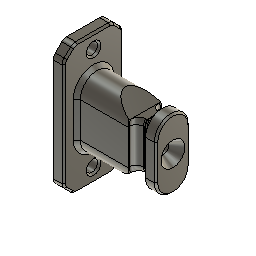
SKADIS_BackSupports (Autodesk Fusion 360 design; units mm, degrees)
Autodesk Fusion 360 part; units mm, degrees
sketch "SlotLayout" plane through (0, 0, 0) normal (1, 0, 0) x (0, 1, 0)
  line L0 (-22.4, 25) -> (-22.4, 15)
  line L1 (82.4, 5) -> (82.4, -5)
  line L2 (-37.6, -5) -> (-37.6, 5)
  line L3 (-80, 5) -> (-80, -5) construction
  line L4 (-97.6, 15) -> (-97.6, 25)
  line L5 (2.4, -5) -> (2.4, 5)
  arc A0 (-77.6, 5) -> (-82.4, 5) centre (-80, 5) ccw
  arc A1 (22.4, 25) -> (17.6, 25) centre (20, 25) ccw
  arc A2 (-97.6, 25) -> (-102.4, 25) centre (-100, 25) ccw
  arc A3 (97.6, 15) -> (102.4, 15) centre (100, 15) ccw
  line L6 (-60, 25) -> (-60, 15) construction
  line L7 (-77.6, -5) -> (-77.6, 5)
  arc A4 (77.6, -5) -> (82.4, -5) centre (80, -5) ccw
  line L8 (-40, 5) -> (-40, -5) construction
  line L9 (-57.6, 15) -> (-57.6, 25)
  line L10 (-62.4, 25) -> (-62.4, 15)
  line L11 (-102.4, 25) -> (-102.4, 15)
  line L12 (97.6, 15) -> (97.6, 25)
  arc A5 (-102.4, 15) -> (-97.6, 15) centre (-100, 15) ccw
  line L13 (20, 25) -> (20, 15) construction
  line L14 (22.4, 25) -> (22.4, 15)
  line L15 (-80, 0) -> (0, 0) construction
  line L16 (62.4, 25) -> (62.4, 15)
  line L17 (42.4, 5) -> (42.4, -5)
  arc A6 (2.5, 5) -> (-2.5, 5) centre (0, 5) ccw
  arc A7 (2.4, 5) -> (-2.4, 5) centre (0, 5) ccw
  line L18 (80, 5) -> (80, -5) construction
  arc A8 (82.4, 5) -> (77.6, 5) centre (80, 5) ccw
  arc A9 (-2.5, -5) -> (2.5, -5) centre (0, -5) ccw
  arc A10 (57.6, 15) -> (62.4, 15) centre (60, 15) ccw
  arc A11 (62.4, 25) -> (57.6, 25) centre (60, 25) ccw
  line L19 (17.6, 15) -> (17.6, 25)
  line L20 (-20, 25) -> (-20, 15) construction
  line L21 (-42.4, 5) -> (-42.4, -5)
  line L22 (60, 25) -> (60, 15) construction
  arc A12 (42.4, 5) -> (37.6, 5) centre (40, 5) ccw
  line L23 (-100, 25) -> (-100, 15) construction
  line L24 (100, 25) -> (100, 15) construction
  arc A13 (-57.6, 25) -> (-62.4, 25) centre (-60, 25) ccw
  arc A14 (37.6, -5) -> (42.4, -5) centre (40, -5) ccw
  line L25 (40, 5) -> (40, -5) construction
  line L26 (-17.6, 15) -> (-17.6, 25)
  arc A15 (-17.6, 25) -> (-22.4, 25) centre (-20, 25) ccw
  line L27 (-82.4, 5) -> (-82.4, -5)
  line L28 (-2.5, 5) -> (-2.5, -5)
  line L29 (-2.4, 5) -> (-2.4, -5)
  line L30 (102.4, 25) -> (102.4, 15)
  arc A16 (17.6, 15) -> (22.4, 15) centre (20, 15) ccw
  arc A17 (-22.4, 15) -> (-17.6, 15) centre (-20, 15) ccw
  line L31 (37.6, -5) -> (37.6, 5)
  line L32 (0, 5) -> (0, -5) construction
  arc A18 (-62.4, 15) -> (-57.6, 15) centre (-60, 15) ccw
  arc A19 (-42.4, -5) -> (-37.6, -5) centre (-40, -5) ccw
  arc A20 (-2.4, -5) -> (2.4, -5) centre (0, -5) ccw
  arc A21 (102.4, 25) -> (97.6, 25) centre (100, 25) ccw
  arc A22 (-82.4, -5) -> (-77.6, -5) centre (-80, -5) ccw
  arc A23 (-37.6, 5) -> (-42.4, 5) centre (-40, 5) ccw
  line L33 (77.6, -5) -> (77.6, 5)
  line L34 (57.6, 15) -> (57.6, 25)
  line L35 (2.5, -5) -> (2.5, 5)
  point P0 (-20, 20)
  point P1 (-40, 0)
  dimension "d9" = -40
  dimension "d10" = 0
  dimension "d255" = 0.1
  dimension "d22" = 10
  dimension "d23" = 2.4
  dimension "d4" = 40
  dimension "d25" = 40
  dimension "d26" = 20
  dimension "d27" = 20
  constraint tangent L27 A22
  constraint tangent L7 A22
  constraint parallel L7 L27
  constraint tangent A0 L7
  constraint tangent A0 L27
  constraint vertical L3
  constraint tangent L21 A19
  constraint tangent L2 A19
  constraint parallel L2 L21
  constraint tangent L2 A23
  constraint tangent L21 A23
  constraint vertical L8
  constraint tangent L29 A20
  constraint tangent L5 A20
  constraint parallel L5 L29
  constraint tangent L5 A7
  constraint tangent A7 L29
  constraint parallel L2 L32
  constraint midpoint L15.start L3
  constraint midpoint L15.end L32
  constraint horizontal L15
  constraint equal L8 L32
  constraint equal L3 L8
  constraint midpoint P1 L8
  constraint coincident P1 L15
  constraint equal A7 A23
  constraint equal A0 A23
  constraint coincident L15.end origin
  constraint symmetric A0.end L1.start L32
  constraint symmetric L1.end L27.end L32
  constraint symmetric L7.start A4.start L32
  constraint symmetric A8.end A0.start L32
  constraint symmetric A4 L32 A22
  constraint symmetric A0 A8 L32
  constraint symmetric L17.start L21.start L32
  constraint symmetric L17.end L21.end L32
  constraint symmetric A14.start L2.start L32
  constraint symmetric A12.end L2.end L32
  constraint symmetric A14 L32 A19
  constraint symmetric A12 L32 A23
  constraint tangent L0 A17
  constraint tangent L26 A17
  constraint parallel L0 L26
  constraint tangent L26 A15
  constraint tangent L0 A15
  constraint vertical L20
  constraint equal L20 L32
  constraint equal A7 A15
  constraint midpoint P0 L20
  constraint symmetric L0.end L14.end L32
  constraint symmetric L26.end A1.end L32
  constraint symmetric L0.start A1.start L32
  constraint symmetric L26.start L19.start L32
  constraint symmetric A1 A15 L32
  constraint symmetric A16 A17 L32
  constraint symmetric A11.end L9.end L32
  constraint symmetric L16.start L10.start L32
  constraint symmetric A11 A13 L32
  constraint symmetric L16.end L10.end L32
  constraint symmetric A10.start L9.start L32
  constraint symmetric A10 L32 A18
  constraint symmetric L12.end L4.end L32
  constraint symmetric L30.start A2.end L32
  constraint symmetric A2 L32 A21
  constraint symmetric A3.end L11.end L32
  constraint symmetric A3.start L4.start L32
  constraint symmetric A3 A5 L32
  measures "d22" distance of A6.centre A9.centre
  measures "d23" radius of A7
  measures "d4" distance of L8 L32
  measures "d25" distance of L3 L8
  measures "d26" horizontal distance of L20.end A6.centre
  measures "d27" vertical distance of P0 L15.end
sketch "VerticalPrintKey" plane through (0, 0, 0) normal (1, 0, 0) x (0, 1, 0)
  line L0 (-2.6, 6.7) -> (2.6, 6.7)
  line L1 (2.6, 6.7) -> (2.6, -6.7)
  line L2 (2.6, -6.7) -> (-2.6, -6.7)
  line L3 (-2.6, -6.7) -> (-2.6, 6.7)
  line L4 (0, 6.7) -> (0, -6.7) construction
  circle A0 centre (0, 0) radius 1.6
  line L5 (2.6, 0) -> (20.8722, 0) construction
  line L6 (20.8722, 0) -> (11.7361, 9.1361) construction
  line L7 (11.7361, 9.1361) -> (11.7361, -9.1361) construction
  line L8 (11.7361, -9.1361) -> (20.8722, 0) construction
  dimension "d18" = 13.4
  dimension "d19" = 5.2
  dimension "d20" = 3.2
  constraint horizontal L0
  constraint vertical L1
  constraint horizontal L2
  constraint vertical L3
  constraint midpoint L0 L4.start
  constraint midpoint L2 L4.end
  constraint midpoint L4 A0.centre
  constraint coincident A0.centre origin
  constraint midpoint L1 L5.start
  constraint perpendicular L1 L5
  constraint perpendicular L5 L7
  constraint perpendicular L6 L8
  constraint midpoint L5 L7
  measures "d18" distance of L4.start L4.end
  measures "d19" distance of L1 L3
  measures "d20" diameter of A0
sketch "HorizontalPrintKey" plane through (0, 0, 0) normal (1, 0, 0) x (0, 1, 0)
  circle A0 centre (0, 0) radius 1.6
  line L0 (2.6, -6.7) -> (-2.6, -6.7)
  line L1 (-2.6, -6.7) -> (-2.6, 6.7)
  line L2 (-2.6, 6.7) -> (2.6, 6.7)
  line L3 (2.6, 6.7) -> (2.6, -6.7)
  line L4 (0, 6.7) -> (0, -6.7) construction
  line L5 (0, 6.7) -> (0, 23.5939) construction
  line L6 (0, 23.5939) -> (-8.4469, 15.1469) construction
  line L7 (-8.4469, 15.1469) -> (8.4469, 15.1469) construction
  line L8 (8.4469, 15.1469) -> (0, 23.5939) construction
  dimension "d21" = 13.4
  dimension "d24" = 5.2
  dimension "d28" = 3.2
  constraint horizontal L2
  constraint vertical L3
  constraint horizontal L0
  constraint vertical L1
  constraint midpoint L4.start L2
  constraint midpoint L4.end L0
  constraint midpoint A0.centre L4
  constraint coincident A0.centre origin
  constraint perpendicular L2 L5
  constraint perpendicular L5 L7
  constraint midpoint L5 L7
  constraint perpendicular L6 L8
  measures "d21" distance of L4.end L4.start
  measures "d24" distance of L1 L3
  measures "d28" diameter of A0
sketch "BaseProfile" plane through (0, 0, 0) normal (1, 0, 0) x (0, 1, 0) in component "SNS_BackSupport"
  line L0 (-4.8, 5) -> (-4.8, -5)
  arc A0 (-4.8, -5) -> (4.8, -5) centre (0, -5) ccw
  line L1 (4.8, -5) -> (4.8, 5)
  arc A1 (4.8, 5) -> (-4.8, 5) centre (0, 5) ccw
  line L2 (0, 5) -> (0, -5) construction
  line L3 (-2.8, -1.6) -> (2.8, -1.6)
  line L4 (-2.8, 1.6166) -> (-2.8, -1.6166)
  circle A2 centre (0, 0) radius 1.6
  line L5 (1.6, 1.6) -> (1.6, -1.6)
  line L6 (-1.6, -1.6) -> (-1.6, 1.6)
  line L7 (-2.8, -1.6166) -> (0, -3.2332)
  line L8 (2.8, 1.6) -> (-2.8, 1.6)
  line L9 (0, 3.2332) -> (-2.8, 1.6166)
  line L10 (2.8, 1.6166) -> (0, 3.2332)
  line L11 (2.8, -1.6166) -> (2.8, 1.6166)
  circle A3 centre (0, 0) radius 2.8 construction
  line L12 (0, -3.2332) -> (2.8, -1.6166)
  line L13 (-2.4, 5) -> (-2.4, -5)
  arc A4 (-2.4, -5) -> (2.4, -5) centre (0, -5) ccw
  line L14 (2.4, -5) -> (2.4, 5)
  arc A5 (2.4, 5) -> (-2.4, 5) centre (0, 5) ccw
  line L15 (0, 5) -> (0, -5) construction
  line L16 (-1.7889, 6.6) -> (1.7889, 6.6)
  line L17 (-1.7889, -6.6) -> (1.7889, -6.6)
  line L18 (8.5, 18.5) -> (-8.5, 18.5)
  line L19 (-8.5, 18.5) -> (-8.5, -18.5)
  line L20 (-8.5, -18.5) -> (8.5, -18.5)
  line L21 (8.5, -18.5) -> (8.5, 18.5)
  line L22 (-8.5, 0) -> (8.5, 0) construction
  line L23 (0, 18.5) -> (0, -18.5) construction
  circle A6 centre (0, -14.5) radius 1.6
  circle A7 centre (0, 14.5) radius 1.6
  dimension "d29" = 4.8
  dimension "d30" = 10
  dimension "d54" = 5.6
  dimension "d34" = 3.2
  dimension "d35" = 2.4
  dimension "d36" = 1.6
  dimension "d37" = 37
  dimension "d38" = 17
  dimension "d72" = 3.2
  dimension "d73" = 4
  dimension "d74" = 4
  constraint tangent L0 A0
  constraint tangent A0 L1
  constraint parallel L0 L1
  constraint tangent L1 A1
  constraint tangent L0 A1
  constraint vertical L2
  constraint midpoint L2 A2.centre
  constraint coincident A2.centre A3.centre
  constraint tangent L4 A3
  constraint vertical L4
  constraint tangent A2 L5
  constraint tangent A2 L6
  constraint coincident L3.start L4
  constraint coincident L3.end L11
  constraint perpendicular L3 L11
  constraint coincident L8.start L11
  constraint coincident L8.end L4
  constraint perpendicular L4 L8
  constraint tangent A2 L8
  constraint tangent L3 A2
  constraint coincident L5.start L8
  constraint perpendicular L5 L8
  constraint coincident L6.start L3
  constraint coincident L6.end L8
  constraint perpendicular L6 L8
  constraint tangent L13 A4
  constraint tangent A4 L14
  constraint parallel L13 L14
  constraint tangent L14 A5
  constraint tangent L13 A5
  constraint coincident A0.centre L2.end
  constraint parallel L2 L15
  constraint coincident A1.centre L2.start
  constraint coincident A5 L16.start
  constraint coincident A5 L16.end
  constraint horizontal L16
  constraint coincident A4 L17.start
  constraint coincident A4 L17.end
  constraint perpendicular L2 L17
  constraint vertical L16.start L17.start
  constraint coincident L5.end L3
  constraint horizontal L18
  constraint vertical L19
  constraint horizontal L20
  constraint vertical L21
  constraint coincident L19 L22.start
  constraint coincident L21 L22.end
  constraint perpendicular L21 L22
  constraint midpoint L21 L22.end
  constraint midpoint L22 A2.centre
  constraint midpoint L18 L23.start
  constraint midpoint L20 L23.end
  constraint coincident L23 A6.centre
  constraint coincident L23 A7.centre
  constraint equal A6 A7
  measures "d29" radius of A1
  measures "d30" distance of A1.centre A0.centre
  measures "d54" diameter of A3
  measures "d34" diameter of A2
  measures "d35" radius of A5
  measures "d36" distance of A1.centre L16
  measures "d37" distance of L18 L20
  measures "d38" distance of L18.start L18.end
  measures "d72" diameter of A6
  measures "d73" distance of L20 A6.centre
  measures "d74" distance of L18 A7.centre
extrude "Extrude1" add sketch "BaseProfile" along normal blind 2.4 contours L3 L6 L8 L13 | L3 L7 L12 L13 L14 | L3 A2 L6 | L8 L9 L10 L13 L14 | L7 L12 L13 A4 L14 L17 | L3 A2 L5 | A2 L6 L8 | L9 L10 L13 L14 A5 L16 | L3 L5 L8 L14 | A2 L5 L8 makes body 1 in component "SNS_BackSupport"
extrude "Extrude2" add sketch "BaseProfile" along normal blind 3 from surface at 2.4 contours L0 A0 L1 A1 | L3 L4 L8 L13 | L3 L4 L7 L13 | L3 L6 L8 L13 | L3 L7 L12 L13 L14 | L4 L8 L9 L13 | L3 A2 L6 | L8 L9 L10 L13 L14 | L7 L12 L13 A4 L14 L17 | L3 A2 L5 | A2 L6 L8 | L9 L10 L13 L14 A5 L16 | L3 L5 L8 L14 | A2 L5 L8 | L3 L11 L12 L14 | A4 L17 | L3 L8 L11 L14 | L8 L10 L11 L14 | A5 L16 bodies 1 in component "SNS_BackSupport"
chamfer "Chamfer1" distance 1.8 distance2 2.8 1 edges at (5.4, -1.4917, 0.5786) measured on face at (5.4, -3.7333, 0) on bodies 1 in component "SNS_BackSupport"
fillet "Fillet1" radius 2 6 edges at (2.4, -2.242, 5.8564) (2.4, -2.4, 0) (2.4, -2.242, -5.8564) (2.4, 2.242, -5.8564) (2.4, 2.4, 0) (2.4, 2.242, 5.8564) on bodies 1 in component "SNS_BackSupport"
chamfer "Chamfer2" distance 0.5 distance2 0.5 4 edges at (5.4, 0, 9.8) (5.4, -4.8, 0) (5.4, 0, -9.8) (5.4, 4.8, 0) measured on face at (5.4, -4.3333, 0) measured on face at (5.4, -4.3333, 0) measured on face at (5.4, -4.3333, 0) measured on face at (5.4, -4.3333, 0) on bodies 1 in component "SNS_BackSupport"
extrude "Extrude3" add 1 faces at (0, 0.0399, -3.8652) along direction (-1, 0, 0) blind 2.4 from surface at 0.2 on bodies 1 bodies 1 makes body 2 in component "SNS_BackSupport"
extrude "Extrude4" add sketch "BaseProfile" against normal blind 17.6 from surface at -2.6 contours L0 A0 L1 A1 | L3 L4 L8 L13 | L3 L4 L7 L13 | L3 L6 L8 L13 | L3 L7 L12 L13 L14 | L4 L8 L9 L13 | L3 A2 L6 | L8 L9 L10 L13 L14 | L7 L12 L13 A4 L14 L17 | L3 A2 L5 | A2 L6 L8 | L9 L10 L13 L14 A5 L16 | L3 L5 L8 L14 | A2 L5 L8 | L3 L11 L12 L14 | A4 L17 | L3 L8 L11 L14 | L8 L10 L11 L14 | A5 L16 bodies 2 in component "SNS_BackSupport"
extrude "Extrude5" add sketch "BaseProfile" along normal blind 3 from surface at -20.2 contours L18 L19 L20 L21 | A6 | A7 bodies 2 in component "SNS_BackSupport"
fillet "Fillet2" radius 2 3 edges at (-2.6, 2.242, 5.8564) (-2.6, 2.4, 0) (-2.6, 2.242, -5.8564) on bodies 2 in component "SNS_BackSupport"
fillet "Fillet2" radius 2 3 edges at (-2.6, -2.242, -5.8564) (-2.6, -2.4, 0) (-2.6, -2.242, 5.8564) on bodies 2 in component "SNS_BackSupport"
sketch "Chamfersides" plane through (0, 0, 0) normal (0, 1, 0) x (1, 0, 0) in component "SNS_BackSupport"
  line L0 (-0.6, -6.6) -> (-2.6, -6.6)
  line L1 (-17.2, -9.8) -> (-17.2, -5)
  line L2 (-17.2, -5) -> (-2.6, -5)
  line L3 (-2.6, -9.8) -> (-2.6, -5)
  line L4 (-2.6, -5) -> (-17.2, -5)
  line L5 (-2.6, -6.6) -> (-8.1426, -9.8)
  line L6 (-8.1426, -9.8) -> (-2.6, -9.8)
  line L7 (0, 0) -> (-32.6284, 0) construction
  line L8 (-2.6, -9.8) -> (-2.6, -6.6)
  line L9 (-2.6, 9.8) -> (-2.6, 6.6)
  line L10 (-2.6, 6.6) -> (-8.1426, 9.8)
  line L11 (-8.1426, 9.8) -> (-2.6, 9.8)
  dimension "d65" = 30
  constraint coincident L0.end L5.start
  constraint perpendicular L3 L6
  constraint coincident L3.start L6.end
  constraint coincident L7.start origin
  constraint horizontal L7
  constraint symmetric L0.end L7 L9.end
  constraint symmetric L5.end L7 L10.end
  constraint symmetric L3.start L7 L9.start
  measures "d65" angle of L5 L6
extrude "Extrude6" cut sketch "Chamfersides" along normal through all and the other way through all bodies 2 in component "SNS_BackSupport"
chamfer "Chamfer4" distance 3 angle 45 4 edges at (-18.7, 8.5, -18.5) (-18.7, -8.5, -18.5) (-18.7, 8.5, 18.5) (-18.7, -8.5, 18.5) on bodies 2 in component "SNS_BackSupport"
fillet "Fillet3" radius 2 8 edges at (-18.7, 5.5, -18.5) (-18.7, 8.5, -15.5) (-18.7, -5.5, -18.5) (-18.7, -8.5, -15.5) (-18.7, 8.5, 15.5) (-18.7, 5.5, 18.5) (-18.7, -5.5, 18.5) (-18.7, -8.5, 15.5) on bodies 2 in component "SNS_BackSupport"
chamfer "Chamfer3" distance 1 angle 45 4 edges at (-17.2, 0, -9.8) (-17.2, 4.8, 0) (-17.2, 0, 9.8) (-17.2, -4.8, 0) on bodies 2 in component "SNS_BackSupport"
chamfer "Chamfer3" distance 0.5 angle 45 16 edges at (-17.2, 7, 17) (-17.2, 8.3478, 15.4369) (-17.2, 8.5, 0) (-17.2, 8.3478, -15.4369) (-17.2, 7, -17) (-17.2, 5.4369, -18.3478) (-17.2, 0, -18.5) (-17.2, -5.4369, -18.3478) (-17.2, -7, -17) (-17.2, -8.3478, -15.4369) (-17.2, -8.5, 0) (-17.2, -8.3478, 15.4369) (-17.2, -7, 17) (-17.2, -5.4369, 18.3478) (-17.2, 0, 18.5) (-17.2, 5.4369, 18.3478) on bodies 2 in component "SNS_BackSupport"
extrude "Extrude7" cut sketch "BaseProfile" against normal through all contours A6 | A7 bodies 2 in component "SNS_BackSupport"
extrude "Extrude8" cut sketch "BaseProfile" along normal up to surface (14.6 mm away) from surface at -20.2 contours L3 L4 L8 L13 | L3 L4 L7 L13 | L3 L6 L8 L13 | L3 L7 L12 L13 L14 | L4 L8 L9 L13 | L3 A2 L6 | L8 L9 L10 L13 L14 | L3 A2 L5 | A2 L6 L8 | L3 L5 L8 L14 | A2 L5 L8 | L3 L11 L12 L14 | L3 L8 L11 L14 | L8 L10 L11 L14 bodies 2 in component "SNS_BackSupport"
extrude "Extrude9" add sketch "BaseProfile" against normal blind 0.2 from surface at -5.6 contours L3 L4 L8 L13 | L3 L6 L8 L13 | L3 L5 L8 L14 | L3 L8 L11 L14 bodies 2 in component "SNS_BackSupport"
extrude "Extrude10" add sketch "BaseProfile" against normal blind 0.4 from surface at -5.6 contours L3 L4 L7 L13 | L3 L7 L12 L13 L14 | L4 L8 L9 L13 | L8 L9 L10 L13 L14 | L3 L11 L12 L14 | L8 L10 L11 L14 bodies 2 in component "SNS_BackSupport"
chamfer "Chamfer5" distance 1 distance2 10 6 edges at (-20.2, -1.4, -2.4249) (-20.2, 2.8, 0) (-20.2, 1.4, 2.4249) (-20.2, -1.4, 2.4249) (-20.2, -2.8, 0) (-20.2, 1.4, -2.4249) measured on face at (-20.2, -6.6, -0.5389) measured on face at (-20.2, -6.6, -0.5389) measured on face at (-20.2, -6.6, -0.5389) measured on face at (-20.2, -6.6, -0.5389) measured on face at (-20.2, -6.6, -0.5389) measured on face at (-20.2, -6.6, -0.5389) on bodies 2 in component "SNS_BackSupport"
chamfer "Chamfer6" distance 0.5 distance2 0.5 2 edges at (-17.2, -1.4917, -13.9214) (-17.2, -1.4917, 15.0786) measured on face at (-17.2, -4.143, -12.9076) measured on face at (-17.2, -4.143, -12.9076) on bodies 2 in component "SNS_BackSupport"
component "SNS_BackSupport" placed x (1, 0, 0) y (0, 1, 0) z (0, 0, 1) at (0, 0, 0)
equation "XY_Tolerance = 0.2 mm"
equation "Z_Tolerance = 0.2 mm"
equation "Wall_Thickness = 0.4 mm"
equation "Layer_Height = 0.2 mm"
equation "M3Hole_wClearance = 3.2 mm"
equation "m3Hole_wSelfTapping = 2.8 mm"
equation "d20 = M3Hole_wClearance"
equation "d28 = M3Hole_wClearance"
equation "d44 = M3Hole_CounterSink"
equation "M3Hole_CounterSink = 1.8 mm"
equation "d56 = -( 20 mm - 2.4 mm )"
equation "d72 = M3Hole_wClearance"
equation "d74 = d73"
equation "d79 = -Layer_Height"
equation "d83 = -Layer_Height * 2"
named bodies: "TopCap", "BackSupport"
